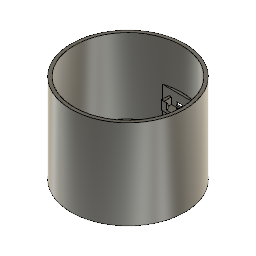
build-button-enclosure (Autodesk Fusion 360 design; units mm, degrees)
Autodesk Fusion 360 part; units mm, degrees
sketch "button-enclosure" plane through (0, 0, 0) normal (0, 0, 1) x (1, 0, 0)
  circle A0 centre (0, 0) radius 35
  circle A1 centre (0, 0) radius 33
  line L0 (-28.6278, 20.1357) -> (28.6278, 20.1357)
  line L1 (33.2711, -10.8643) -> (-33.2711, -10.8643)
  line L2 (-15.4609, 31.4) -> (15.4609, 31.4)
  line L3 (0, 0) -> (0, 35) construction
  point P0 (0, 35)
  dimension "d24" = 70
  dimension "d25" = 66
  dimension "d32" = 31
  dimension "d36" = 3.6
  constraint coincident A0.centre A1.centre
  constraint concentric A0 A1
  constraint horizontal L0
  constraint horizontal L1
  constraint coincident A0 L0.start
  constraint coincident A0 L1.end
  constraint coincident A0 L1.start
  constraint coincident A0 L0.end
  constraint coincident A0 L2.end
  constraint horizontal L2
  constraint coincident A0 L2.start
  constraint coincident A0 P0
  constraint perpendicular L0 L3
  constraint coincident P0 L3.end
  measures "d24" diameter of A0
  measures "d25" diameter of A1
  measures "d32" distance of L0 L1
  measures "d36" distance of L2 P0
extrude "Extrude9" add sketch "button-enclosure" along normal blind 55 contours A0 A1 L0 L1 | A0 A1 L0 L2 | A0 A1 L1 | A0 A1 L2 | A0 A1 L0 L1 | A0 A1 L0 L2
extrude "Extrude8" add sketch "button-enclosure" along normal blind 3
extrude "Extrude10" add sketch "button-enclosure" along normal blind 9 contours A1 L0 L2 | A1 L1 | A1 L2
extrude "Extrude11" add sketch "button-enclosure" along normal blind 30 contours A1 L2
ref_plane "WorkPlane3" through (0, 31.4, 19.5) normal (0, -1, 0) x (1, 0, 0)
ref_plane "WorkPlane4" through (0, 32.4, 19.5) normal (0, -1, 0) x (1, 0, 0)
sketch "flat-surface" plane through (0, 32.4, 32) normal (0, -1, 0) x (1, 0, 0)
  line L0 (8.5, -23.8701) -> (-8.5, -23.8701)
  line L1 (-11.5, -20.8701) -> (-11.5, -5.8701)
  line L2 (-8.5, -2.8701) -> (8.5, -2.8701)
  line L3 (11.5, -5.8701) -> (11.5, -20.8701)
  arc A0 (11.5, -5.8701) -> (8.5, -2.8701) centre (8.5, -5.8701) ccw
  arc A1 (-8.5, -2.8701) -> (-11.5, -5.8701) centre (-8.5, -5.8701) ccw
  arc A2 (8.5, -23.8701) -> (11.5, -20.8701) centre (8.5, -20.8701) ccw
  arc A3 (-11.5, -20.8701) -> (-8.5, -23.8701) centre (-8.5, -20.8701) ccw
  line L4 (35, -32) -> (-35, -32)
  line L5 (0, -32) -> (0, 8.7435) construction
  line L6 (3.5688, -18.24) -> (-3.59, -18.24)
  line L7 (-4.59, -19.24) -> (-4.59, -19.2996)
  line L8 (-2.09, -21.7996) -> (2.0688, -21.7996)
  line L9 (4.5688, -19.2996) -> (4.5688, -19.24)
  arc A4 (2.0688, -21.7996) -> (4.5688, -19.2996) centre (2.0688, -19.2996) ccw
  arc A5 (-4.59, -19.2996) -> (-2.09, -21.7996) centre (-2.09, -19.2996) ccw
  arc A6 (4.5688, -19.24) -> (3.5688, -18.24) centre (3.5688, -19.24) ccw
  arc A7 (-3.59, -18.24) -> (-4.59, -19.24) centre (-3.59, -19.24) ccw
  line L10 (-1.85, -9.0168) -> (1.85, -9.0168)
  line L11 (1.85, -9.0168) -> (1.85, -7.0168)
  line L12 (1.85, -7.0168) -> (-1.85, -7.0168)
  line L13 (-1.85, -7.0168) -> (-1.85, -9.0168)
  line L14 (-1.85, -9.0168) -> (1.85, -7.0168) construction
  line L15 (1.85, -9.0168) -> (-1.85, -7.0168) construction
  line L16 (4.675, -6.0168) -> (-4.675, -6.0168)
  line L17 (-4.675, -6.0168) -> (-4.675, -10.0168)
  line L18 (-4.675, -10.0168) -> (4.675, -10.0168)
  line L19 (4.675, -10.0168) -> (4.675, -6.0168)
  line L20 (4.675, -6.0168) -> (-4.675, -10.0168) construction
  line L21 (-4.675, -6.0168) -> (4.675, -10.0168) construction
  line L22 (-4.675, -6.0168) -> (-6.175, -6.0168)
  line L23 (-6.175, -6.0168) -> (-6.175, -11.5168)
  line L24 (-6.175, -11.5168) -> (6.175, -11.5168)
  line L25 (6.175, -11.5168) -> (6.175, -6.0168)
  line L26 (6.175, -6.0168) -> (4.675, -6.0168)
  line L27 (-3.175, -6.0168) -> (-3.175, -10.0168)
  line L28 (3.175, -6.0168) -> (3.175, -10.0168)
  point P0 (0, -32)
  point P1 (0, -2.8701)
  point P2 (4.5688, -18.24)
  point P3 (0, -8.0168)
  point P4 (0, -8.0168)
  dimension "d43" = 3
  dimension "d44" = 3
  dimension "d45" = 3
  dimension "d46" = 3
  dimension "d49" = 21
  dimension "d50" = 23
  dimension "d51" = 2.5
  dimension "d54" = 1
  dimension "d55" = 1
  dimension "d78" = 3.7
  dimension "d79" = 2
  dimension "d82" = 9.35
  dimension "d83" = 4
  dimension "d84" = 1.5
  dimension "d85" = 1.5
  dimension "d86" = 1.5
  dimension "d87" = 1.5
  dimension "d88" = 1.5
  constraint horizontal L0
  constraint vertical L1
  constraint horizontal L2
  constraint vertical L3
  constraint tangent L2 A0
  constraint tangent L3 A0
  constraint tangent L1 A1
  constraint tangent L2 A1
  constraint tangent L0 A2
  constraint tangent L3 A2
  constraint tangent L0 A3
  constraint tangent L1 A3
  constraint coincident P0 L5.start
  constraint perpendicular L4 L5
  constraint midpoint L2 P1
  constraint coincident L5 P1
  constraint horizontal L6
  constraint vertical L7
  constraint horizontal L8
  constraint vertical L9
  constraint tangent L8 A4
  constraint tangent L9 A4
  constraint tangent L7 A5
  constraint tangent L8 A5
  constraint equal A4 A5
  constraint tangent L6 A6
  constraint tangent L9 A6
  constraint tangent L6 A7
  constraint tangent L7 A7
  constraint perpendicular L10 L11
  constraint parallel L10 L12
  constraint parallel L11 L13
  constraint horizontal L10
  constraint coincident L14 P4
  constraint coincident L15 P4
  constraint coincident L5 P4
  constraint perpendicular L16 L17
  constraint parallel L16 L18
  constraint parallel L17 L19
  constraint horizontal L16
  constraint coincident L20 P4
  constraint coincident L21 P4
  constraint coincident P4 P3
  constraint perpendicular L17 L22
  constraint perpendicular L16 L23
  constraint perpendicular L17 L24
  constraint perpendicular L16 L25
  constraint perpendicular L19 L26
  constraint coincident L16 L27.start
  constraint coincident L18 L27.end
  constraint perpendicular L18 L27
  constraint coincident L16 L28.start
  constraint coincident L18 L28.end
  constraint perpendicular L18 L28
  measures "d43" radius of A0
  measures "d44" radius of A1
  measures "d45" radius of A2
  measures "d46" radius of A3
  measures "d49" distance of L0 L2
  measures "d50" distance of L1 L3
  measures "d51" radius of A4
  measures "d54" radius of A6
  measures "d55" radius of A7
  measures "d78" distance of L11.end L12.end
  measures "d79" distance of L10.end L11.end
  measures "d82" distance of L17.end L18.end
  measures "d83" distance of L16.end L17.end
  measures "d84" distance of L17 L23
  measures "d85" distance of L18 L24
  measures "d86" distance of L19 L25
  measures "d87" distance of L17 L27
  measures "d88" distance of L19 L28
ref_plane "WorkPlane6" through (-0.0106, 27.8, 11.9802) normal (0, -1, 0) x (1, 0, 0)
extrude "Extrude19" cut sketch "flat-surface" along normal blind 4 contours L10 L11 L12 L13
extrude "Extrude12" cut sketch "flat-surface" against normal blind 17 contours L0 L1 L2 L3 A0 A1 A2 A3 | L6 L7 L8 L9 A4 A5 A6 A7 | L10 L11 L12 L13 | L16 L18 L19 L28 | L17 L18 L19 L22 L23 L24 L25 L26 | L16 L18 L27 L28 | L16 L17 L18 L27
extrude "Extrude13" cut sketch "flat-surface" along normal blind 4 contours L6 L7 L8 L9 A4 A5 A6 A7
ref_plane "WorkPlane5" through (0, 0, 105) normal (0, 0, 1) x (1, 0, 0)
sketch "feather-mounting-holes" plane through (0, 0, 9) normal (0, 0, 1) x (-1, 0, 0)
  line L0 (-10.1509, -31.4) -> (10.1509, -31.4)
  arc A0 (10.1509, -31.4) -> (26.1449, -20.1357) centre (0, 0) ccw
  line L1 (26.1449, -20.1357) -> (-26.1449, -20.1357)
  arc A1 (-26.1449, -20.1357) -> (-10.1509, -31.4) centre (0, 0) ccw
  circle A2 centre (8.89, -28.6978) radius 1.275
  circle A3 centre (-8.89, -28.653) radius 1.275
  circle A4 centre (8.89, 17.1572) radius 1.275
  circle A5 centre (-8.89, 17.0677) radius 1.275
  dimension "d72" = 2.55
  dimension "d73" = 2.55
  dimension "d74" = 2.55
  dimension "d75" = 2.55
  measures "d72" diameter of A2
  measures "d73" diameter of A3
  measures "d74" diameter of A4
  measures "d75" diameter of A5
extrude "Extrude18" cut sketch "feather-mounting-holes" against normal blind 8 contours A2 | A3 | A4 | A5
extrude "Extrude20" add sketch "flat-surface" along normal blind 4.6 contours L17 L18 L19 L22 L23 L24 L25 L26
sketch "switch-holder-lip" plane through (0, 27.8, 32) normal (0, -1, 0) x (1, 0, 0)
  line L0 (-3.175, -6.0168) -> (-3.175, -10.0168)
  line L1 (-6.175, -6.0168) -> (-3.175, -6.0168)
  line L2 (-3.175, -10.0168) -> (3.175, -10.0168)
  line L3 (4.675, -6.0168) -> (-4.675, -6.0168)
  line L4 (3.175, -10.0168) -> (3.175, -6.0168)
  line L5 (-6.175, -11.5168) -> (6.175, -11.5168)
  line L6 (6.175, -6.0168) -> (6.175, -11.5168)
  line L7 (-6.175, -11.5168) -> (-6.175, -6.0168)
  line L8 (4.675, -6.0168) -> (6.175, -6.0168)
  point P0 (-6.175, -6.0168)
  point P1 (-3.175, -6.0168)
  point P2 (3.175, -10.0168)
  point P3 (3.175, -6.0168)
  point P4 (6.175, -6.0168)
  point P5 (6.175, -11.5168)
  constraint coincident P0 L1.start
  constraint coincident P1 L0.start
  constraint coincident L0.end L2.start
  constraint coincident P2 L2.end
  constraint coincident P3 L4.end
  constraint coincident P4 L6.start
  constraint coincident P5 L5.end
  constraint coincident L5.start L7.start
  constraint coincident L3.start L8.start
extrude "Extrude21" add sketch "switch-holder-lip" along normal blind 1 contours L0 L1 L2 L3 L4 L5 L6 L7 L8
fillet "Fillet3" radius 2 2 edges at (3.925, 27.8, 25.9832) (-3.925, 27.8, 25.9832)
chamfer "Chamfer1" distance 4.6 angle 45 1 edges at (0, 31.4, 20.4832)
named bodies: "enclosure"
